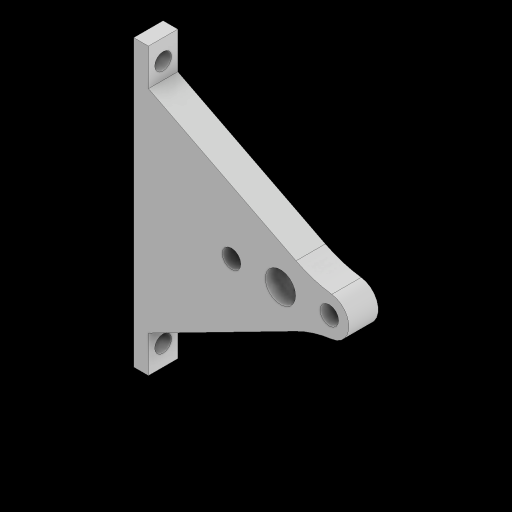
# Autodesk Inventor part: TransmissonCoreMount
Saved by Autodesk Inventor 2024.1 (Build 281209000, 209)
## iProperties
Created: 2025-05-07
Part Number: TransmissonCoreMount
Material: Generic
Document SubType Name: Modeling
Designer: Teddy
Density: 1 g/cm^3
Appearance: Default
Author: Teddy
Autodesk Inventor part; units mm, degrees
ref_plane "YZ Plane" through (0, 0, 0) normal (1, 0, 0) x (0, 1, 0)
ref_plane "XZ Plane" through (0, 0, 0) normal (0, 1, 0) x (-1, 0, 0)
ref_plane "Work Plane1" through (0, 0, 0) normal (0, 0, 1) x (1, 0, 0)
sketch "Sketch1" plane through (0, 0, 0) normal (0, 0, 1) x (1, 0, 0)
  circle A0 centre (0, 12.7) radius 2.1844 projected
  line L0 (12.7, -0.9398) -> (12.7, -62.4078) projected
  line L1 (0, 12.7) -> (50.8, 12.7) construction
  circle A1 centre (50.8, 12.7) radius 3.937
  circle A2 centre (50.8, 12.7) radius 8.89
  line L2 (12.7, -16.7386) -> (11.1125, -16.7386) construction
  line L3 (12.7, -21.3614) -> (11.1125, -21.3614) construction
  line L4 (12.7, 46.7614) -> (11.1125, 46.7614) construction
  line L5 (12.7, 42.1386) -> (11.1125, 42.1386) construction
  line L6 (54.8432, 20.6174) -> (16.51, 40.193)
  line L7 (54.8432, 4.7826) -> (16.51, -14.793)
  line L8 (12.7, 42.1386) -> (12.7, -16.7386)
  line L9 (16.51, 40.193) -> (16.51, 49.7586)
  line L10 (16.51, 49.7586) -> (12.7, 49.7586)
  line L11 (12.7, 49.7586) -> (12.7, 42.1386)
  line L12 (16.51, 40.193) -> (16.51, -14.793) construction
  line L13 (16.51, -24.3586) -> (12.7, -24.3586)
  line L14 (12.7, -16.7386) -> (12.7, -24.3586)
  line L15 (16.51, -24.3586) -> (16.51, -14.793)
  line L16 (16.51, 40.193) -> (12.7, 42.1386) construction
  line L17 (16.51, -14.793) -> (12.7, -16.7386) construction
  circle A3 centre (38.1, 12.7) radius 2.413
  circle A4 centre (63.5, 12.7) radius 2.413
  circle A5 centre (63.5, 12.7) radius 5.08
  arc A6 (54.8432, 20.6174) -> (64.1482, 17.7385) centre (67.7772, 45.945) ccw
  arc A7 (64.1482, 7.6615) -> (54.8432, 4.7826) centre (67.7772, -20.545) ccw
  point P0 (0, 0)
  dimension "d0" = 50.8
  dimension "d1" = 7.874
  dimension "d2" = 17.78
  dimension "d3" = 3.81
  dimension "d4" = 7.62
  dimension "d5" = 7.62
  dimension "d10" = 4.826
  dimension "d11" = 4.826
  dimension "d12" = 12.7
  dimension "d13" = 12.7
  dimension "d14" = 10.16
  constraints: 26 end point, 8 point on circle, 8 tangent, 7 centre point, 5 point on line, 3 coincident, 3 perpendicular, 2 collinear, 1 horizontal, 1 horizontal alignment, 1 parallel, 1 vertical
  measures "d0" distance of L1.start L1.end
  measures "d1" diameter of A1
  measures "d2" diameter of A2
  measures "d3" distance between parallel lines of L0 L12
  measures "d4" distance between parallel lines of L2 L13
  measures "d5" distance between parallel lines of L5 L10
  measures "d10" diameter of A3
  measures "d11" diameter of A4
  measures "d12" distance of L1.end A4.centre
  measures "d13" distance of L1.end A3.centre
  measures "d14" diameter of A5
extrude "Extrusion1" add sketch "Sketch1" along normal blind 7.62 contours L8 L11 L10 L9 L6 A2 L7 L15 L13 L0 | A2 A5 | A2 A5 A7 | A6 A5 A2 | A5 A2 | A2 A5
sketch "Sketch2" plane through (16.51, -24.3586, 0) normal (1, 0, 0) x (0, 0, -1)
  circle A0 centre (7.9375, 5.3086) radius 2.1844 projected
  circle A1 centre (7.9375, 68.8086) radius 2.1844 projected
  circle A2 centre (-3.81, 5.3086) radius 2.1844
  circle A3 centre (-3.81, 68.8086) radius 2.1844
  line L0 (0, 0) -> (-7.62, 0) projected
  point P0 (0, 24.3586)
  point P1 (-3.81, 0)
  constraints: 2 centre point, 2 equal radius, 2 horizontal alignment, 2 vertical alignment, 1 midpoint
extrude "Extrusion2" cut sketch "Sketch2" against normal blind 6.35 contours A2 | A3
body "Solid1"
